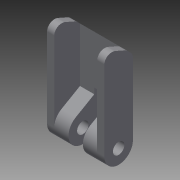
# Autodesk Inventor part: LegV5
Saved by Autodesk Inventor 2014 (Build 180170000, 170)
## iProperties
Created: 2014-04-27
Part Number: LegV5
Material: Generic
Document SubType Name: Modeling
Designer: Max
Density: 1 g/cm^3
Appearance: Default
Author: Max
Autodesk Inventor part; units mm, degrees
ref_plane "YZ Plane" through (0, 0, 0) normal (1, 0, 0) x (0, 1, 0)
ref_plane "XZ Plane" through (0, 0, 0) normal (0, 1, 0) x (-1, 0, 0)
ref_plane "XY Plane" through (0, 0, 0) normal (0, 0, 1) x (1, 0, 0)
sketch "Sketch1" plane through (0, 0, 0) normal (1, 0, 0) x (0, 1, 0)
  circle A0 centre (0, 0) radius 2.54
  circle A1 centre (0, 0) radius 6.35
  line L0 (0, 6.35) -> (40.2531, 6.35)
  line L1 (40.2531, 6.35) -> (40.2531, -6.35)
  line L2 (40.2531, -6.35) -> (0, -6.35)
  line L3 (40.2531, 6.35) -> (34.5987, -6.35)
  line L4 (35.1642, -5.08) -> (3.81, -5.08)
  line L5 (5.4993, 3.175) -> (10.2653, -5.08)
  line L6 (12.8053, -5.08) -> (12.8053, -6.35)
  dimension "d0" = 5.08
  dimension "d1" = 12.7
  dimension "d2" = 66
  dimension "d12" = 3.175
  dimension "d13" = 1.27
  dimension "d16" = 2.54
  constraints: 14 end point, 5 point on line, 4 point on circle, 3 tangent, 2 centre point, 2 coincident, 2 horizontal, 2 perpendicular, 1 parallel
  measures "d0" diameter of A0
  measures "d1" diameter of A1
  measures "d2" angle of L2 L3
  measures "d12" vertical distance of point (0, 0) L5.start
  measures "d13" distance between parallel lines of L2 L4
  measures "d16" distance from line of L5.end L6
extrude "Extrusion1" add sketch "Sketch1" along normal mid plane 25.4 contours A1 | A1 L5 L4 | A1 L0 L3 L4 L5 | L4 L6 L2 A1 | L4 L3 L2 L6
chamfer "Chamfer1" distance 1.5875 distance2 3.175 1 edges at (0, 34.5987, -6.35) measured on face at (4.2333, 23.0658, -6.35)
chamfer "Chamfer2" distance 4.7625 distance2 1.5875 1 edges at (0, 40.2531, 6.35) measured on face at (4.2333, 38.7988, 3.0835)
fillet "Fillet1" radius 3.175 4 edges at (0, 38.6656, 6.35) (0, 38.316, 1.9992) (0, 35.8901, -3.4495) (0, 33.0112, -6.35)
extrude "Extrusion2" cut sketch "Sketch1" along normal mid plane 19.05 contours A1 L0 L3 L4 L5
extrude "Extrusion3" cut sketch "Sketch1" along normal mid plane 6.35 contours A1 | A1 L5 L4 | L4 L6 L2 A1
equation "\"d12\" = 0.25 * d1"
body "Solid1"
